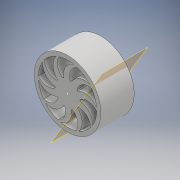
# Autodesk Inventor part: Колесо
Saved by Autodesk Inventor 2018 (Build 220112000, 112)
## iProperties
Created: 2019-08-24
Part Number: Колесо
Material: Типовые
Document SubType Name: Modeling
Designer: KV33_HP1
Density: 1 g/cm^3
Appearance: По умолчанию
Author: KV33_HP1
Autodesk Inventor part; units mm, degrees
ref_plane "YZ Plane" through (0, 0, 0) normal (1, 0, 0) x (0, 1, 0)
ref_plane "XZ Plane" through (0, 0, 0) normal (0, 1, 0) x (-1, 0, 0)
ref_plane "XY Plane" through (0, 0, 0) normal (0, 0, 1) x (1, 0, 0)
sketch "Эскиз1" plane through (0, 0, 0) normal (0, 1, 0) x (-1, 0, 0)
  circle A0 centre (0, 0) radius 20
  circle A1 centre (0, 0) radius 17.5
  dimension "d0" = 40
  dimension "d1" = 35
  constraints: 2 centre point, 2 coincident
  measures "d0" diameter of A0
  measures "d1" diameter of A1
extrude "Выдавливание1" add sketch "Эскиз1" along normal blind 20
sketch "Эскиз2" plane through (0, 0, 0) normal (0, -1, 0) x (1, 0, 0)
  circle A0 centre (0, 0) radius 7.5
  dimension "d5" = 15
  constraints: 1 centre point, 1 coincident
  measures "d5" diameter of A0
extrude "Выдавливание2" add sketch "Эскиз2" against normal blind 25
sketch "Эскиз3" plane through (0, 0, 0) normal (0, -1, 0) x (1, 0, 0)
  arc A0 (6.4343, -3.8535) -> (7.5, 0) centre (0, 0) ccw
  circle A1 centre (0, 0) radius 17.5 projected
  arc A2 (13.9071, -10.6227) -> (14.995, -9.0222) centre (0, 0) ccw
  circle A3 centre (0, 0) radius 7.5 projected
  arc A4 (14.995, -9.0222) -> (7.5, 0) centre (6.4343, -8.5096) ccw
  arc A5 (13.9071, -10.6227) -> (6.4343, -3.8535) centre (6.8631, -10.8895) ccw
  arc A6 (17.4343, 1.5147) -> (6.0676, 4.4084) centre (10.2073, -3.1024) ccw
  arc A7 (7.4705, 0.6644) -> (6.0676, 4.4084) centre (0, 0) ccw
  arc A8 (17.495, -0.4196) -> (7.4705, 0.6644) centre (11.9531, -4.7757) ccw
  arc A9 (17.495, -0.4196) -> (17.4343, 1.5147) centre (0, 0) ccw
  arc A10 (13.2143, 11.4731) -> (2.3176, 7.1329) centre (10.0814, 3.4898) ccw
  arc A11 (5.6532, 4.9286) -> (2.3176, 7.1329) centre (0, 0) ccw
  arc A12 (14.4004, 9.9438) -> (5.6532, 4.9286) centre (12.4773, 3.1622) ccw
  arc A13 (14.4004, 9.9438) -> (13.2143, 11.4731) centre (0, 0) ccw
  arc A14 (3.9469, 17.0491) -> (-2.3176, 7.1329) centre (6.1048, 8.749) ccw
  arc A15 (1.6766, 7.3102) -> (-2.3176, 7.1329) centre (0, 0) ccw
  arc A16 (5.8053, 16.509) -> (1.6766, 7.3102) centre (8.2357, 9.8923) ccw
  arc A17 (5.8053, 16.509) -> (3.9469, 17.0491) centre (0, 0) ccw
  arc A18 (-6.8281, 16.1129) -> (-6.0676, 4.4084) centre (-0.2037, 10.6664) ccw
  arc A19 (-2.9404, 6.8996) -> (-6.0676, 4.4084) centre (0, 0) ccw
  arc A20 (-5.0072, 16.7684) -> (-2.9404, 6.8996) centre (0.8483, 12.8438) ccw
  arc A21 (-5.0072, 16.7684) -> (-6.8281, 16.1129) centre (0, 0) ccw
  arc A22 (-14.995, 9.0222) -> (-7.5, 0) centre (-6.4343, 8.5096) ccw
  arc A23 (-6.4343, 3.8535) -> (-7.5, 0) centre (0, 0) ccw
  arc A24 (-13.9071, 10.6227) -> (-6.4343, 3.8535) centre (-6.8631, 10.8895) ccw
  arc A25 (-13.9071, 10.6227) -> (-14.995, 9.0222) centre (0, 0) ccw
  arc A26 (-17.4343, -1.5147) -> (-6.0676, -4.4084) centre (-10.2073, 3.1024) ccw
  arc A27 (-7.4705, -0.6644) -> (-6.0676, -4.4084) centre (0, 0) ccw
  arc A28 (-17.495, 0.4196) -> (-7.4705, -0.6644) centre (-11.9531, 4.7757) ccw
  arc A29 (-17.495, 0.4196) -> (-17.4343, -1.5147) centre (0, 0) ccw
  arc A30 (-13.2143, -11.4731) -> (-2.3176, -7.1329) centre (-10.0814, -3.4898) ccw
  arc A31 (-5.6532, -4.9286) -> (-2.3176, -7.1329) centre (0, 0) ccw
  arc A32 (-14.4004, -9.9438) -> (-5.6532, -4.9286) centre (-12.4773, -3.1622) ccw
  arc A33 (-14.4004, -9.9438) -> (-13.2143, -11.4731) centre (0, 0) ccw
  arc A34 (-3.9469, -17.0491) -> (2.3176, -7.1329) centre (-6.1048, -8.749) ccw
  arc A35 (-1.6766, -7.3102) -> (2.3176, -7.1329) centre (0, 0) ccw
  arc A36 (-5.8053, -16.509) -> (-1.6766, -7.3102) centre (-8.2357, -9.8923) ccw
  arc A37 (-5.8053, -16.509) -> (-3.9469, -17.0491) centre (0, 0) ccw
  arc A38 (6.8281, -16.1129) -> (6.0676, -4.4084) centre (0.2037, -10.6664) ccw
  arc A39 (2.9404, -6.8996) -> (6.0676, -4.4084) centre (0, 0) ccw
  arc A40 (5.0072, -16.7684) -> (2.9404, -6.8996) centre (-0.8483, -12.8438) ccw
  arc A41 (5.0072, -16.7684) -> (6.8281, -16.1129) centre (0, 0) ccw
  dimension "d10" = 360
  constraints: 82 point on circle, 40 centre point, 2 coincident, 121 other
extrude "Выдавливание3" add sketch "Эскиз3" against normal blind 10 contours A0 A4 A1 A5 | A38 A1 A40 A3 | A3 A6 A1 A8 | A34 A1 A36 A3 | A3 A10 A1 A12 | A30 A1 A32 A3 | A3 A14 A1 A16 | A26 A1 A28 A3 | A3 A18 A1 A20 | A22 A1 A24 A3
sketch "Эскиз5" plane through (0, 25, 0) normal (0, 1, 0) x (1, 0, 0)
  circle A0 centre (0, 0) radius 2.1
  dimension "d14" = 4.2
  constraints: 1 centre point, 1 coincident
  measures "d14" diameter of A0
extrude "Выдавливание4" cut sketch "Эскиз5" against normal blind 15
ref_plane "РабПлоскость1" through (6.4343, 0, -3.8535) normal (0.8579, 0, -0.5138) x (0, 1, 0)
sketch "Эскиз6" plane through (6.4343, 0, -3.8535) normal (0.8579, 0, -0.5138) x (0, 1, 0)
  line L0 (25, -7.5) -> (25, 7.5) projected
  line L1 (25, 0) -> (19, 0)
  circle A0 centre (19, 0) radius 1.4
  point P0 (0, 0)
  dimension "d17" = 6
  dimension "d18" = 2.8
  constraints: 2 end point, 1 centre point, 1 coincident, 1 horizontal, 1 midpoint
  measures "d17" distance of L1.start L1.end
  measures "d18" diameter of A0
extrude "Выдавливание5" cut sketch "Эскиз6" against normal blind 15
sketch "Эскиз7" plane through (0, 0, 0) normal (0, -1, 0) x (1, 0, 0)
  point P0 (0, 0)
